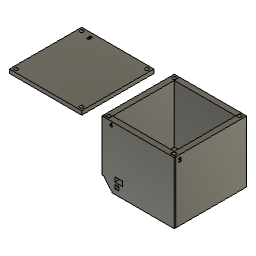
timecube_v3_finished (Autodesk Fusion 360 design; units mm, degrees)
Autodesk Fusion 360 part; units mm, degrees
note: some values were not read from the file. Chosen so that the rebuilt part matches the saved one: which bodies a step acts on.
sketch "Szkic1" plane through (0, 0, 0) normal (0, 0, 1) x (1, 0, 0)
  line L0 (-40, -40) -> (40, -40)
  line L1 (40, -40) -> (40, 40)
  line L2 (40, 40) -> (-40, 40)
  line L3 (-40, 40) -> (-40, -40)
  constraint horizontal L0
  constraint vertical L1
  constraint horizontal L2
  constraint vertical L3
extrude "Wyciągnięcie proste1" add sketch "Szkic1" along normal blind 5 makes body 1
copy_body "Kopiuj-wklej bryły1" bodies 1 makes body 2
move_body "Przesuń1" bodies 2 to x (0, 0, 1) y (0, 1, 0) z (-1, 0, 0) at (-40.0538, 0.9669, 40)
move_body "Przesuń2" bodies 2 to x (1, 0, 0) y (0, 1, 0) z (0, 0, 1) at (0.0835, -0.5312, 0)
copy_body "Kopiuj-wklej bryły2" bodies 2 makes body 3
move_body "Przesuń3" bodies 3 to x (0, 1, 0) y (-1, 0, 0) z (0, 0, 1) at (0.3461, 1.3934, 0)
move_body "Przesuń4" bodies 2 to x (1, 0, 0) y (0, 1, 0) z (0, 0, 1) at (-47.9337, 0.9875, -22.9426)
move_body "Przesuń5" bodies 3 to x (1, 0, 0) y (0, 1, 0) z (0, 0, 1) at (0, -27.0109, 1.9748)
move_body "Wyrównaj1" bodies 1 to x (1, 0, 0) y (0, 1, 0) z (0, 0, 1) at (0, -25.5878, 1.9748)
extrude "Wyciągnięcie proste2" add 1 faces at (-89.5706, -38.5768, 3.7241) along direction (0, -1, 0) blind 10 on bodies 2 bodies 2
move_body "Wyrównaj2" bodies 2 to x (1, 0, 0) y (0, 1, 0) z (0, 0, 1) at (47.904, 0, 24.9174)
move_body "Wyrównaj3" bodies 2 to x (1, 0, 0) y (0, 1, 0) z (0, 0, 1) at (-0.0896, -22.0109, 0)
copy_body "Kopiuj-wklej bryły3" bodies 2 makes body 4
move_body "Przesuń6" bodies 4 to x (1, 0, 0) y (0, 1, 0) z (0, 0, 1) at (85, 0, 0)
copy_body "Kopiuj-wklej bryły4" bodies 3 makes body 5
move_body "Przesuń7" bodies 5 to x (1, 0, 0) y (0, 1, 0) z (0, 0, 1) at (0, 85, 0)
combine "Kombinacja1" operation add target body 1 tool bodies 3 2 keep tools
sketch "Szkic4" plane through (-45.0896, 0, 0) normal (-1, 0, 0) x (0, -1, 0)
  line L0 (-19.4122, 1.9748) -> (70.5878, 1.9748)
  line L1 (70.5878, 1.9748) -> (70.5878, 81.9748)
  line L2 (70.5878, 81.9748) -> (-19.4122, 81.9748)
  line L3 (-19.4122, 81.9748) -> (-19.4122, 1.9748)
  line L4 (58.1813, 1.9748) -> (70.5878, 15.6535)
  line L5 (70.5878, 1.9748, 0) -> (70.5878, 1.9748, -85)
  line L6 (70.5878, 1.9748, -11.8154) -> (70.5878, 15.6535, 0)
  line L7 (58.1813, 1.9748, 0) -> (70.5878, 1.9748, -11.8154)
  constraint coincident L0 L4.start
  constraint coincident L1 L4.end
sketch "Szkic4 (curves on the plane with normal -0.6139, -0.5847, -0.5303 at 32.9705 mm)" plane through (-65.3313, -19.2774, -17.4845) normal (-0.613935, -0.584686, -0.530308) x (0, -0.671823, 0.740711)
  line L0 (40.5503, -25.6433) -> (59.0172, -25.6433)
  line L1 (48.8853, -40.6117) -> (59.0172, -25.6433)
  line L2 (40.5503, -25.6433) -> (48.8853, -40.6117)
extrude "Wyciągnięcie proste3" cut sketch "Szkic4 (curves on the plane with normal -0.6139, -0.5847, -0.5303 at 32.9705 mm)" along normal blind 140 bodies 1 2 3
extrude "Wyciągnięcie proste4" cut sketch "Szkic4 (curves on the plane with normal -0.6139, -0.5847, -0.5303 at 32.9705 mm)" against normal blind 100 bodies 1 2 3
sketch "Szkic5" plane through (0, -70.5878, 0) normal (0, -1, 0) x (1, 0, 0)
  line L0 (-40.0896, 9.865) -> (-33.2741, 1.9748)
  line L1 (-33.2741, 1.9748) -> (39.9104, 1.9748)
  line L2 (39.9104, 1.9748) -> (39.9104, 81.9748)
  line L3 (39.9104, 81.9748) -> (-40.0896, 81.9748)
  line L4 (-40.0896, 81.9748) -> (-40.0896, 9.865)
  line L5 (-30.2673, 13.3958) -> (-25.2673, 13.3958)
  line L6 (-25.2673, 13.3958) -> (-25.2673, 8.3958)
  line L7 (-25.2673, 8.3958) -> (-30.2673, 8.3958)
  line L8 (-30.2673, 8.3958) -> (-30.2673, 13.3958)
  dimension "d9" = 5
  dimension "d10" = 5
  constraint horizontal L5
  constraint vertical L6
  constraint horizontal L7
  constraint vertical L8
  measures "d9" distance of L5.start L5.end
  measures "d10" distance of L5.start L7.end
extrude "Wyciągnięcie proste5" cut sketch "Szkic5" against normal blind 30 contours L5 L6 L7 L8 bodies 1 3
sketch "Szkic6" plane through (0, -70.5878, 0) normal (0, -1, 0) x (1, 0, 0)
  line L0 (-25.2673, 13.3958) -> (-25.2673, 8.3958)
  line L1 (-25.2673, 8.3958) -> (-30.2673, 8.3958)
  line L2 (-30.2673, 8.3958) -> (-30.2673, 13.3958)
  line L3 (-30.2673, 13.3958) -> (-25.2673, 13.3958)
  line L4 (-40.0896, 9.865) -> (-33.2741, 1.9748)
  line L5 (-33.2741, 1.9748) -> (39.9104, 1.9748)
  line L6 (39.9104, 1.9748) -> (39.9104, 81.9748)
  line L7 (39.9104, 81.9748) -> (-40.0896, 81.9748)
  line L8 (-40.0896, 81.9748) -> (-40.0896, 9.865)
  line L9 (-30.2673, 15.856) -> (-24.2673, 15.856)
  line L10 (-24.2673, 15.856) -> (-24.2673, 21.856)
  line L11 (-24.2673, 21.856) -> (-30.2673, 21.856)
  line L12 (-30.2673, 21.856) -> (-30.2673, 15.856)
  dimension "d13" = 6
  dimension "d14" = 6
  constraint horizontal L9
  constraint vertical L10
  constraint horizontal L11
  constraint vertical L12
  measures "d13" distance of L9.start L9.end
  measures "d14" distance of L9.start L11.end
extrude "Wyciągnięcie proste6" cut sketch "Szkic6" against normal blind 30 contours L9 L10 L11 L12 bodies 1 3
sketch "Szkic7" plane through (0, 19.4122, 0) normal (0, 1, 0) x (-1, 0, 0)
  line L0 (-39.9104, 1.9748) -> (40.0896, 1.9748)
  line L1 (40.0896, 1.9748) -> (40.0896, 81.9748)
  line L2 (40.0896, 81.9748) -> (-39.9104, 81.9748)
  line L3 (-39.9104, 81.9748) -> (-39.9104, 1.9748)
  line L4 (-44.9104, 81.9748, -90) -> (45.0182, 81.9748, -90)
  line L5 (45.0182, 81.9748, -90) -> (45.0182, 0, -90)
  line L6 (45.0182, 0, -90) -> (-44.9104, 0, -90)
  line L7 (-44.9104, 0, -90) -> (-44.9104, 81.9748, -90)
  point P0 (-44.9104, 81.9748)
sketch "Szkic8" plane through (0, 0, 81.9748) normal (0, 0, 1) x (-1, 0, 0)
  line L0 (-44.9104, 70.5878) -> (-44.9104, -19.4122)
  line L1 (-44.9104, -19.4122) -> (-39.9104, -19.4122)
  line L2 (-39.9104, -19.4122) -> (-39.9104, 70.5878)
  line L3 (-39.9104, 70.5878) -> (-44.9104, 70.5878)
  line L4 (-44.9104, 70.5878) -> (45.2681, 70.5878)
  line L5 (45.2681, 70.5878) -> (45.2681, -19.9712)
  line L6 (45.2681, -19.9712) -> (-44.9104, -19.9712)
  line L7 (-44.9104, -19.9712) -> (-44.9104, 70.5878)
  constraint horizontal L4
  constraint vertical L5
  constraint horizontal L6
  constraint vertical L7
  constraint coincident L0.start L3.end
extrude "Wyciągnięcie proste7" add sketch "Szkic8" along normal blind 10 separate body makes body 6
extrude "Wyciągnięcie proste8" cut 1 faces at (13.1842, -10.4014, 91.9748) along direction (0, 0, -1) blind 5 on bodies 6 bodies 6
move_body "Przesuń8" bodies 6 to x (1, 0, 0) y (0, 1, 0) z (0, 0, 1) at (115.0461, 25.7468, 0)
sketch "Szkic9" plane through (0, 0, 81.9748) normal (0, 0, 1) x (-1, 0, 0)
  line L0 (40.0896, 70.5878) -> (40.0896, -19.4122)
  line L1 (40.0896, -19.4122) -> (45.0896, -19.4122)
  line L2 (45.0896, -19.4122) -> (45.0896, 70.5878)
  line L3 (45.0896, 70.5878) -> (40.0896, 70.5878)
split "Podział1" by plane through (-40.0896, -20.5878, 41.9748) normal (1, 0, 0) bodies 1 makes body 7 at (13.3035, -38.2337, 1.9748)
move_body "Przesuń9" bodies 1 to x (1, 0, 0) y (0, 1, 0) z (0, 0, 1) at (-40.2935, -0.1474, 0)
delete_body "Usuń bryłę1" bodies 1
split "Podział2" by plane through (-0.0896, -65.5878, 41.9748) normal (0, 1, 0) bodies 7 makes body 8 at (13.3035, -38.2337, 1.9748)
delete_body "Usuń bryłę2" bodies 7
sketch "Szkic10" plane through (0, 0, 81.9748) normal (0, 0, 1) x (-1, 0, 0)
  line L0 (40.0896, 70.5878) -> (40.0896, -19.4122)
  line L1 (40.0896, -19.4122) -> (45.0896, -19.4122)
  line L2 (45.0896, -19.4122) -> (45.0896, 70.5878)
  line L3 (45.0896, 70.5878) -> (40.0896, 70.5878)
  line L4 (-39.9104, -14.4122) -> (40.0896, -14.4122)
  circle A0 centre (42.5896, -16.9122) radius 2.5
  line L5 (-44.9104, -19.4122) -> (-44.9104, 70.5878)
  line L6 (-44.9104, -19.4122) -> (-39.9104, -19.4122)
  line L7 (-39.9104, -19.4122) -> (-39.9104, 70.5878)
  circle A1 centre (-42.4104, -16.9122) radius 2.5
  line L8 (-44.9104, 70.5878) -> (-39.9104, 70.5878)
  circle A2 centre (-42.4104, 68.0878) radius 2.5
  circle A3 centre (42.5896, 68.0878) radius 2.5
  constraint tangent L2 A0
  constraint tangent L1 A0
  constraint tangent L4 A0
  constraint tangent L5 A1
  constraint tangent L6 A1
  constraint tangent L7 A1
  constraint tangent L5 A2
  constraint tangent L8 A2
  constraint tangent L7 A2
  constraint tangent L2 A3
  constraint tangent L3 A3
  constraint tangent L0 A3
delete_body "Usuń bryłę3" bodies 6
sketch "Szkic11" plane through (0, 0, 81.9748) normal (0, 0, 1) x (-1, 0, 0)
  line L0 (-44.9104, 70.5878) -> (45.0896, 70.5878)
  line L1 (45.0896, 70.5878) -> (45.0896, -19.4122)
  line L2 (45.0896, -19.4122) -> (-44.9104, -19.4122)
  line L3 (-44.9104, -19.4122) -> (-44.9104, 70.5878)
  point P0 (-44.9104, 70.5878)
  point P1 (45.0896, -19.4122)
  constraint horizontal L0
  constraint vertical L1
  constraint horizontal L2
  constraint vertical L3
  constraint coincident P1 L1.end
  constraint coincident P0 L0.start
extrude "Wyciągnięcie proste9" add sketch "Szkic11" along normal blind 5 separate body makes body 9
move_body "Przesuń10" bodies 9 to x (1, 0, 0) y (0, 1, 0) z (0, 0, 1) at (0, 0, -5)
hole "Otwór1" at (42.4104, 16.9122, 81.9748) at (-42.5896, 16.9122, 81.9748) at (-42.5896, -68.0878, 81.9748) at (42.4104, -68.0878, 81.9748) direction (0, 0, -1) diameter 4.6 depth 5 tip angle 180 bodies 2 4 9
move_body "Przesuń11" bodies 9 to x (1, 0, 0) y (0, 1, 0) z (0, 0, 1) at (0, 0, 5)
sketch "Szkic12" plane through (0, 0, 86.9748) normal (0, 0, 1) x (-1, 0, 0)
  circle A0 centre (42.5896, 68.0878) radius 2.3
  circle A1 centre (-42.4104, -16.9122) radius 2.3
  circle A2 centre (42.5896, -16.9122) radius 2.3
  circle A3 centre (-42.4104, 68.0878) radius 2.3
  line L0 (-44.9104, -19.4122) -> (45.0896, -19.4122)
  line L1 (45.0896, -19.4122) -> (45.0896, 70.5878)
  line L2 (45.0896, 70.5878) -> (-44.9104, 70.5878)
  line L3 (-44.9104, 70.5878) -> (-44.9104, -19.4122)
  line L4 (35.2523, -10) -> (25, -10) construction
  line L5 (25, -10) -> (25, -19.4122) construction
  line L6 (25, -19.4122) -> (35.2523, -19.4122) construction
  line L7 (35.2523, -19.4122) -> (35.2523, -10) construction
  dimension "d26" = 5
  text T0 "5" font "Arial" height 5 align centre middle in box 10.2523 x 9.4122 at (35.2523, -10) x (-1, 0) y (0, -1) spacing 1
  constraint coincident L0
extrude "Wyciągnięcie proste10" cut sketch "Szkic12" against normal blind 1 text T0 bodies 9
sketch "Szkic13" plane through (0, -70.5878, 0) normal (0, -1, 0) x (1, 0, 0)
  line L0 (-24.2673, 15.856) -> (-30.2673, 15.856)
  line L1 (-30.2673, 15.856) -> (-30.2673, 21.856)
  line L2 (-30.2673, 21.856) -> (-24.2673, 21.856)
  line L3 (-24.2673, 21.856) -> (-24.2673, 15.856)
  line L4 (-25.2673, 13.3958) -> (-25.2673, 8.3958)
  line L5 (-25.2673, 8.3958) -> (-30.2673, 8.3958)
  line L6 (-30.2673, 8.3958) -> (-30.2673, 13.3958)
  line L7 (-30.2673, 13.3958) -> (-25.2673, 13.3958)
  line L8 (-40.0896, 9.865) -> (-33.2741, 1.9748)
  line L9 (-33.2741, 1.9748) -> (39.9104, 1.9748)
  line L10 (39.9104, 1.9748) -> (39.9104, 81.9748)
  line L11 (39.9104, 81.9748) -> (-40.0896, 81.9748)
  line L12 (-40.0896, 81.9748) -> (-40.0896, 9.865)
  line L13 (-40.0896, 73.8434) -> (-30.7147, 73.8434) construction
  line L14 (-30.7147, 73.8434) -> (-30.7147, 81.9748) construction
  line L15 (-30.7147, 81.9748) -> (-40.0896, 81.9748) construction
  line L16 (-40.0896, 81.9748) -> (-40.0896, 73.8434) construction
  dimension "d29" = 5
  text T0 "4" font "Arial" height 5 align centre middle in box 9.3748 x 8.1315 at (-40.0896, 73.8434) x (1, 0) y (0, 1) spacing 1
  constraint coincident L11.end
sketch "Szkic14" plane through (44.9104, 0, 0) normal (1, 0, 0) x (0, 1, 0)
  line L0 (-70.5878, 1.9748) -> (19.4122, 1.9748)
  line L1 (19.4122, 1.9748) -> (19.4122, 81.9748)
  line L2 (19.4122, 81.9748) -> (-70.5878, 81.9748)
  line L3 (-70.5878, 81.9748) -> (-70.5878, 1.9748)
  line L4 (-70.5878, 70) -> (-60, 70) construction
  line L5 (-60, 70) -> (-60, 81.9748) construction
  line L6 (-60, 81.9748) -> (-70.5878, 81.9748) construction
  line L7 (-70.5878, 81.9748) -> (-70.5878, 70) construction
  dimension "d30" = 5
  text T0 "3" font "Arial" height 5 align centre middle in box 10.5878 x 11.9748 at (-70.5878, 70) x (1, 0) y (0, 1) spacing 1
  constraint coincident L2.end
sketch "Szkic15" plane through (0, 19.4122, 0) normal (0, 1, 0) x (-1, 0, 0)
  line L0 (-39.9104, 1.9748) -> (40.0896, 1.9748)
  line L1 (40.0896, 1.9748) -> (40.0896, 81.9748)
  line L2 (40.0896, 81.9748) -> (-39.9104, 81.9748)
  line L3 (-39.9104, 81.9748) -> (-39.9104, 1.9748)
  line L4 (-39.9104, 72.5273) -> (-30.593, 72.5273) construction
  line L5 (-30.593, 72.5273) -> (-30.593, 81.9748) construction
  line L6 (-30.593, 81.9748) -> (-39.9104, 81.9748) construction
  line L7 (-39.9104, 81.9748) -> (-39.9104, 72.5273) construction
  dimension "d31" = 5
  text T0 "2" font "Arial" height 5 align centre middle in box 9.3174 x 9.4475 at (-39.9104, 72.5273) x (1, 0) y (0, 1) spacing 1
  constraint coincident L2.end
sketch "Szkic16" plane through (-45.0896, 0, 0) normal (-1, 0, 0) x (0, -1, 0)
  line L0 (58.1813, 1.9748) -> (70.5878, 15.6535)
  line L1 (70.5878, 15.6535) -> (70.5878, 81.9748)
  line L2 (70.5878, 81.9748) -> (-19.4122, 81.9748)
  line L3 (-19.4122, 81.9748) -> (-19.4122, 1.9748)
  line L4 (-19.4122, 1.9748) -> (58.1813, 1.9748)
  line L5 (-19.4122, 70.8287) -> (-8.3667, 70.8287) construction
  line L6 (-8.3667, 70.8287) -> (-8.3667, 81.9748) construction
  line L7 (-8.3667, 81.9748) -> (-19.4122, 81.9748) construction
  line L8 (-19.4122, 81.9748) -> (-19.4122, 70.8287) construction
  dimension "d32" = 5
  text T0 "1" font "Arial" height 5 align centre middle in box 11.0456 x 11.1461 at (-19.4122, 70.8287) x (1, 0) y (0, 1) spacing 1
  constraint coincident L2.end
sketch "Szkic17" plane through (0, 0, 1.9748) normal (0, 0, -1) x (1, 0, 0)
  line L0 (40, 65.5878) -> (-38.0359, 65.5878)
  line L1 (-38.0359, 65.5878) -> (-40, 63.5255)
  line L2 (-40, 63.5255) -> (-40, -14.4122)
  line L3 (-40, -14.4122) -> (40, -14.4122)
  line L4 (40, -14.4122) -> (40, 65.5878)
  line L5 (-40, 55) -> (-29.2383, 55) construction
  line L6 (-29.2383, 55) -> (-29.2383, 65.5878) construction
  line L7 (-29.2383, 65.5878) -> (-40, 65.5878) construction
  line L8 (-40, 65.5878) -> (-40, 55) construction
  dimension "d33" = 5
  text T0 "6" font "Arial" height 5 align centre middle in box 10.7617 x 10.5878 at (-40, 55) x (1, 0) y (0, 1) spacing 1
  constraint coincident L0
  constraint coincident L2
extrude "Wyciągnięcie proste11" cut sketch "Szkic17" against normal blind 1 text T0 bodies 8
extrude "Wyciągnięcie proste12" cut sketch "Szkic15" against normal blind 1 text T0 bodies 5
extrude "Wyciągnięcie proste13" cut sketch "Szkic14" against normal blind 1 text T0 bodies 4
extrude "Wyciągnięcie proste14" cut sketch "Szkic13" against normal blind 1 text T0 bodies 3
extrude "Wyciągnięcie proste15" cut sketch "Szkic16" against normal blind 1 text T0 bodies 2
extrude "Wyciągnięcie proste16" add 1 faces at (-45.0896, -8.6002, 25.9505) along direction (-1, 0, 0) blind 2 separate body on bodies 2 makes body 10
combine "Kombinacja2" operation add target body 2 tool bodies 10
extrude "Wyciągnięcie proste17" add 1 faces at (-44.0896, -70.5878, 59.8677) along direction (0, -1, 0) blind 2 separate body on bodies 2 makes body 11
extrude "Wyciągnięcie proste18" add 1 faces at (18.5178, -70.5878, 35.2685) along direction (0, -1, 0) blind 2 separate body on bodies 3 makes body 12
extrude "Wyciągnięcie proste19" add 1 faces at (43.2438, -70.5878, 28.6415) along direction (0, -1, 0) blind 2 separate body on bodies 4 makes body 13
extrude "Wyciągnięcie proste20" add 1 faces at (44.9104, -8.3837, 52.6638) along direction (1, 0, 0) blind 2 separate body on bodies 4 makes body 14
extrude "Wyciągnięcie proste21" add 1 faces at (44.9104, -71.9211, 28.6415) along direction (1, 0, 0) blind 2 separate body on bodies 13 makes body 15
extrude "Wyciągnięcie proste22" add 1 faces at (-42.4229, 19.4122, 55.3082) along direction (0, 1, 0) blind 2 separate body on bodies 2 makes body 16
extrude "Wyciągnięcie proste23" add 1 faces at (-15.5267, 19.4122, 52.9002) along direction (0, 1, 0) blind 2 separate body on bodies 5 makes body 17
combine "Kombinacja3" operation add target body 3 tool bodies 12 11 13 15
combine "Kombinacja4" operation add target body 14 tool bodies 4
extrude "Wyciągnięcie proste24" add 1 faces at (44.5771, 19.4122, 28.6415) along direction (0, 1, 0) blind 2 separate body on bodies 14 makes body 18
combine "Kombinacja5" operation add target body 14 tool bodies 18
combine "Kombinacja6" operation add target body 2 tool bodies 16
combine "Kombinacja7" operation add target body 5 tool bodies 17
move_body "Przesuń12" bodies 9 to x (1, 0, 0) y (0, 1, 0) z (0, 0, 1) at (-108.0371, -12.334, 0)
extrude "Wyciągnięcie proste25" add 1 faces at (-93.1267, -82.9218, 83.6415) along direction (0, -1, 0) blind 2 on bodies 9 bodies 9
extrude "Wyciągnięcie proste26" add 1 faces at (-63.1267, -54.2551, 83.6415) along direction (1, 0, 0) blind 2 on bodies 9 bodies 9
extrude "Wyciągnięcie proste27" add 1 faces at (-91.7933, 7.0782, 85.3082) along direction (0, 1, 0) blind 2 on bodies 9 bodies 9
extrude "Wyciągnięcie proste28" add 1 faces at (-153.1267, -22.2551, 85.3082) along direction (-1, 0, 0) blind 2 on bodies 9 bodies 9
extrude "Wyciągnięcie proste29" cut 1 faces at (-24.2673, -67.9211, 17.856) along direction (1, 0, 0) blind 4 on bodies 3 bodies 3
named bodies: "z_6", "x_1", "y_4", "x_3", "y_2", "z_5", "z_6 (1)"
